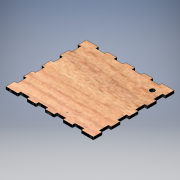
# Autodesk Inventor part: BaseModule
Saved by Autodesk Inventor 2019.4 (Build 234330000, 330)
## iProperties
Created: 2020-06-30
Part Number: BaseModule
Material: Wood (Birch)
Document SubType Name: Modeling
Designer: wimva
Density: 0.55 g/cm^3
Appearance: Birch - Natural Polished
Author: wimva
Autodesk Inventor part; units mm, degrees
ref_plane "YZ Plane" through (0, 0, 0) normal (1, 0, 0) x (0, 1, 0)
ref_plane "XZ Plane" through (0, 0, 0) normal (0, 1, 0) x (-1, 0, 0)
ref_plane "XY Plane" through (0, 0, 0) normal (0, 0, 1) x (1, 0, 0)
sketch "Rectangle" plane through (0, 0, 0) normal (0, 1, 0) x (-1, 0, 0)
  line L0 (-48.26, -44.5) -> (48.26, -44.5)
  line L1 (48.26, -44.5) -> (48.26, 44.5)
  line L2 (48.26, 44.5) -> (-48.26, 44.5)
  line L3 (-48.26, 44.5) -> (-48.26, -44.5)
  line L4 (-48.26, -44.5) -> (48.26, 44.5) construction
  line L5 (48.26, -44.5) -> (-48.26, 44.5) construction
  point P0 (0, 0)
  dimension "d12" = 96.52
  dimension "d13" = 89
  constraints: 12 end point, 2 midpoint, 2 parallel, 1 horizontal, 1 perpendicular
  measures "d12" distance of L2.end L1.end
  measures "d13" distance of L2.end L0.start
extrude "Extrusion1" add sketch "Rectangle" along normal blind 3
sketch "Sketch3" plane through (0, 3, 0) normal (0, 1, 0) x (1, 0, 0)
  line L0 (48.26, 44.5) -> (-48.26, 44.5) construction
  line L1 (-15, 44.5) -> (-5, 44.5)
  line L2 (-5, 44.5) -> (-5, 41.5)
  line L3 (-5, 41.5) -> (-15, 41.5)
  line L4 (-15, 41.5) -> (-15, 44.5)
  line L5 (0, 62.3) -> (0, -62.3) construction
  point P0 (0, 0)
  dimension "d14" = 10
  dimension "d16" = 3
  dimension "d22" = 5
  constraints: 8 end point, 2 parallel, 1 horizontal, 1 perpendicular, 1 point on line
  measures "d14" distance of L2.end L3.end
  measures "d16" distance of L1.end L2.end
  measures "d22" distance between parallel lines of L5 L2
extrude "Extrusion3" cut sketch "Sketch3" against normal through all
pattern_linear "Rectangular Pattern2" count 2 spacing 20 along (-1, 0, 0) count 2 spacing 40 along (1, 0, 0) of "Extrusion3"
mirror "Mirror2" about plane through (0, 0, 0) normal (0, 0, 1) of "Extrusion3", "Rectangular Pattern2"
sketch "Sketch4" plane through (0, 3, 0) normal (0, 1, 0) x (1, 0, 0)
  line L0 (67.564, 0) -> (-67.564, 0) construction
  line L1 (-48.26, 44.5) -> (-48.26, -44.5) construction
  line L2 (-48.26, 15) -> (-45.26, 15)
  line L3 (-45.26, 15) -> (-45.26, 5)
  line L4 (-45.26, 5) -> (-48.26, 5)
  line L5 (-48.26, 5) -> (-48.26, 15)
  point P0 (0, 0)
  dimension "d23" = 3
  dimension "d24" = 10
  dimension "d25" = 5
  constraints: 8 end point, 2 parallel, 1 horizontal, 1 perpendicular, 1 point on line
  measures "d23" distance of L3.end L4.end
  measures "d24" distance of L2.end L3.end
  measures "d25" distance between parallel lines of L0 L4
extrude "Extrusion4" cut sketch "Sketch4" against normal through all
pattern_linear "Rectangular Pattern3" count 2 spacing 20 along (0, 0, -1) count 2 spacing 40 along (0, 0, 1) of "Extrusion4"
mirror "Mirror4" about plane through (0, 0, 0) normal (1, 0, 0) of "Extrusion4", "Rectangular Pattern3"
sketch "Sketch5" plane through (0, 3, 0) normal (0, 1, 0) x (1, 0, 0)
  line L0 (48.26, 35) -> (48.26, 44.5) construction
  line L1 (48.26, 44.5) -> (35, 44.5) construction
  point P0 (0, 0)
  point P1 (36.26, 32.5)
  dimension "d31" = 12
  dimension "d32" = 12
  measures "d31" distance from line of L0 point (36.26, 32.5)
  measures "d32" distance from line of point (36.26, 32.5) L1
hole "Hole1" at (36.26, 3, -32.5) direction (0, -1, 0) diameter 5 end through all
equation "\"d12\" = Module_Width"
equation "\"d13\" = Module_Height"
equation "\"d2\" = Module_Case_Thickness"
equation "\"d14\" = Module_Case_SlotWidth"
equation "\"d16\" = Module_Case_SlotDepth"
equation "\"d22\" = 0.5 * Module_Case_SlotWidth"
equation "\"d21\" = 2 * Module_Case_SlotWidth"
equation "\"d42\" = 4 * Module_Case_SlotWidth"
equation "\"d23\" = Module_Case_SlotDepth"
equation "\"d24\" = Module_Case_SlotWidth"
equation "\"d25\" = 0.5 * Module_Case_SlotWidth"
equation "\"d30\" = 2 * Module_Case_SlotWidth"
equation "\"d45\" = 4 * Module_Case_SlotWidth"
equation "\"d33\" = Module_StatusIndicatorDiameter"
equation "\"RackWidth\" = 482.6"
equation "\"U\" = 44.5"
equation "\"Module_Connector_Width\" = 6"
equation "\"Module_Case_SlotWidth\" = 10"
equation "\"Module_Case_SlotDepth\" = 3"
equation "\"Module_Back_Thickness\" = 5"
equation "\"Module_Connector_Depth\" = 4"
equation "\"Module_Height\" = 89"
equation "\"Module_Width\" = 96.52"
equation "\"Module_Case_Thickness\" = 3"
equation "\"Module_StatusIndicatorDiameter\" = 5"
equation "\"Module_Case_BottomSlotDepth\" = 5"
body "Solid1"
